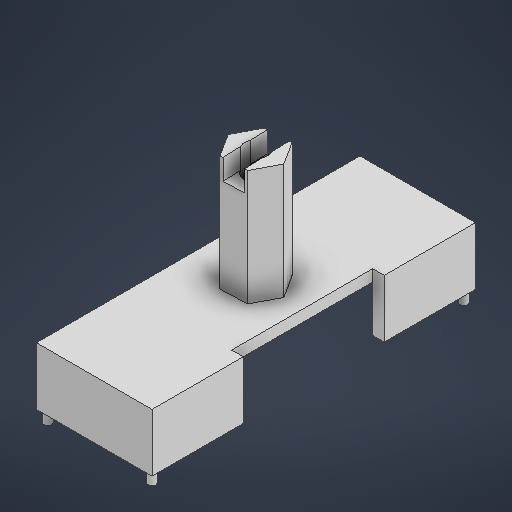
# Autodesk Inventor part: Caja_Antena
Saved by Autodesk Inventor 2026 (Build 300175000, 175)
## iProperties
Created: 2025-11-03
Part Number: Caja_Antena
Material: Generic
Document SubType Name: Modeling
Designer: Nicolás De Bruijn
Density: 1 g/cm^3
Appearance: Default
Author: Nicolás De Bruijn
Autodesk Inventor part; units mm, degrees
ref_plane "YZ Plane" through (0, 0, 0) normal (1, 0, 0) x (0, 1, 0)
ref_plane "XZ Plane" through (0, 0, 0) normal (0, 1, 0) x (-1, 0, 0)
ref_plane "XY Plane" through (0, 0, 0) normal (0, 0, 1) x (1, 0, 0)
sketch "Sketch1" plane through (0, 0, 0) normal (0, 1, 0) x (-1, 0, 0)
  point P0 (0, 0)
sketch "Sketch2" plane through (0, 0, 0) normal (0, 1, 0) x (-1, 0, 0)
  line L0 (11.0402, 14.5) -> (-38.9598, 14.5)
  line L1 (-38.9598, -125.5) -> (11.0402, -125.5)
  line L2 (11.0402, -125.5) -> (11.0402, 14.5)
  line L3 (-38.9598, -25) -> (-33.9598, -25)
  line L4 (-38.9598, -86) -> (-33.9598, -86)
  line L5 (-38.9598, 14.5) -> (-38.9598, -25)
  line L6 (-38.9598, -86) -> (-38.9598, -125.5)
  line L7 (-33.9598, -25) -> (-33.9598, 9.5)
  line L8 (-33.9598, 9.5) -> (6.0402, 9.5)
  line L9 (6.0402, 9.5) -> (6.0402, -120.5)
  line L10 (6.0402, -120.5) -> (-33.9598, -120.5)
  line L11 (-33.9598, -120.5) -> (-33.9598, -86)
  point P0 (0, 0)
  dimension "d0" = 50
  dimension "d1" = 140
  dimension "d2" = 5
  dimension "d3" = 39.5
  dimension "d4" = 39.5
  dimension "d5" = 34.5
  dimension "d6" = 40
  dimension "d7" = 130
  constraints: 24 end point, 7 perpendicular, 4 parallel, 2 horizontal, 1 point on line, 1 vertical
  measures "d0" distance of L1.end L1.start
  measures "d1" distance of L1.start L0.end
  measures "d2" distance of L3.start L3.end
  measures "d3" distance between parallel lines of L0 L3
  measures "d4" distance between parallel lines of L1 L4
  measures "d5" distance of L3.end L7.end
  measures "d6" distance of L7.end L8.end
  measures "d7" distance of L8.end L9.end
extrude "Extrusion1" add sketch "Sketch2" along normal blind 20
sketch "Sketch3" plane through (0, 20, 0) normal (0, 1, 0) x (1, 0, 0)
  line L0 (-11.0402, 125.5) -> (-11.0402, -14.5) projected
  line L1 (38.9598, 125.5) -> (-11.0402, 125.5) projected
  line L2 (-11.0402, -14.5) -> (38.9598, -14.5)
  line L3 (38.9598, 125.5) -> (-11.0402, 125.5)
  line L4 (-11.0402, 125.5) -> (-11.0402, -14.5)
  line L5 (33.9598, 86) -> (38.9598, 86) projected
  line L6 (38.9598, 25) -> (33.9598, 25) projected
  line L7 (33.9598, 25) -> (33.9598, -9.5) projected
  line L8 (33.9598, 25) -> (33.9598, 86)
  line L9 (38.9598, -14.5) -> (38.9598, 25)
  line L10 (38.9598, 86) -> (38.9598, 125.5)
  point P0 (0, 0)
  constraints: 14 end point, 3 parallel, 2 perpendicular, 1 horizontal, 1 vertical
extrude "Extrusion2" add sketch "Sketch3" along normal blind 5
sketch "Sketch4" plane through (0, 25, 0) normal (0, 1, 0) x (1, 0, 0)
  circle A0 centre (13.9598, 55.5) radius 5
  line L0 (-11.0402, -14.5) -> (38.9598, -14.5) projected
  line L1 (38.9598, 86) -> (38.9598, 125.5) projected
  point P0 (0, 0)
  dimension "d12" = 10
  dimension "d13" = 70
  dimension "d14" = 25
  constraints: 1 centre point
  measures "d12" diameter of A0
  measures "d13" distance from line of L0 A0.centre
  measures "d14" distance from line of L1 A0.centre
extrude "Extrusion3" cut sketch "Sketch4" against normal blind 5
sketch "Sketch5" plane through (0, 0, 0) normal (0, -1, 0) x (1, 0, 0)
  circle A0 centre (36.4598, 12) radius 1.6
  line L0 (38.9598, 14.5) -> (38.9598, -25) projected
  line L1 (-11.0402, 14.5) -> (38.9598, 14.5) projected
  circle A1 centre (36.4598, -123) radius 1.6
  line L2 (38.9598, -125.5) -> (-11.0402, -125.5) projected
  line L3 (38.9598, -86) -> (38.9598, -125.5) projected
  circle A2 centre (-8.5402, -123) radius 1.6
  line L4 (-11.0402, -125.5) -> (-11.0402, 14.5) projected
  circle A3 centre (-8.5402, 12) radius 1.6
  point P0 (0, 0)
  dimension "d17" = 3.2
  dimension "d18" = 2.5
  dimension "d19" = 2.5
  dimension "d20" = 3.2
  dimension "d21" = 2.5
  dimension "d22" = 2.5
  dimension "d23" = 3.2
  dimension "d24" = 2.5
  dimension "d25" = 2.5
  dimension "d26" = 3.2
  dimension "d27" = 2.5
  dimension "d28" = 2.5
  constraints: 4 centre point
  measures "d17" diameter of A0
  measures "d18" distance from line of L0 A0.centre
  measures "d19" distance from line of A0.centre L1
  measures "d20" diameter of A1
  measures "d21" distance from line of L2 A1.centre
  measures "d22" distance from line of L3 A1.centre
  measures "d23" diameter of A2
  measures "d24" distance from line of L2 A2.centre
  measures "d25" distance from line of L4 A2.centre
  measures "d26" diameter of A3
  measures "d27" distance from line of A3.centre L1
  measures "d28" distance from line of L4 A3.centre
extrude "Extrusion4" add sketch "Sketch5" along normal blind 5
sketch "Sketch6" plane through (0, 25, 0) normal (0, 1, 0) x (1, 0, 0)
  circle A0 centre (13.9598, 55.5) radius 5 projected
  line L0 (8.5818, 45.2818) -> (2.4216, 55.0484)
  line L1 (2.4216, 55.0484) -> (7.7996, 65.2665)
  line L2 (7.7996, 65.2665) -> (19.3378, 65.7182)
  line L3 (19.3378, 65.7182) -> (25.498, 55.9516)
  line L4 (25.498, 55.9516) -> (20.12, 45.7335)
  line L5 (20.12, 45.7335) -> (8.5818, 45.2818)
  point P0 (0, 0)
  dimension "d31" = 10
  constraints: 12 end point, 1 coincident, 13 other
  measures "d31" distance from line of L1 point (13.96, 55.5)
extrude "Extrusion5" add sketch "Sketch6" along normal blind 50
sketch "Sketch7" plane through (20.12, 25, -45.7335) normal (0.0391109, 0, 0.9992349) x (0.9992349, 0, -0.0391109)
  point P0 (-21.8933, -25)
sketch "Sketch8" plane through (20.12, 25, -45.7335) normal (0.0391109, 0, 0.9992349) x (0.9992349, 0, -0.0391109)
  line L0 (-10.7735, 50) -> (-0.7735, 50) projected
  line L1 (-10.273, 50) -> (-1.273, 50)
  line L2 (-1.273, 50) -> (-1.273, 41)
  line L3 (-1.273, 41) -> (-10.273, 41)
  line L4 (-10.273, 41) -> (-10.273, 50)
  line L5 (0, 0) -> (0, 50) projected
  line L6 (-11.547, 0) -> (-11.547, 50) projected
  point P0 (-21.8933, -25)
  point P1 (-1.273, 50)
  dimension "d34" = 9
  dimension "d35" = 9
  dimension "d36" = 1.273
  dimension "d37" = 1.274
  constraints: 8 end point, 2 parallel, 1 horizontal, 1 perpendicular, 1 point on line
  measures "d34" distance of L2.end L3.end
  measures "d35" distance of L1.end L2.end
  measures "d36" distance between parallel lines of L5 L2
  measures "d37" distance between parallel lines of L4 L6
extrude "Extrusion6" cut sketch "Sketch8" against normal through all
body "Solid1"
